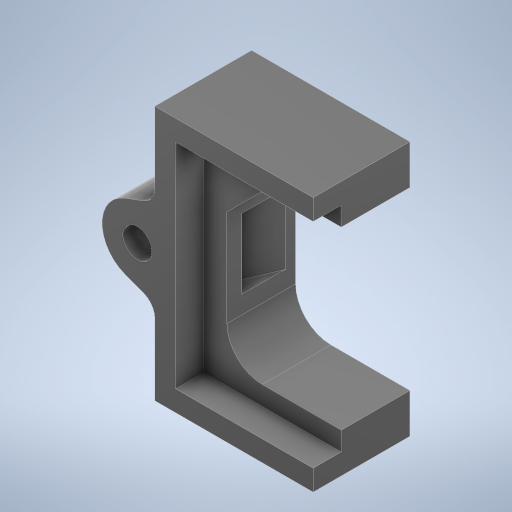
# Autodesk Inventor part: power_signal_socket_fixed2
Saved by Autodesk Inventor 2023 (Build 270158000, 158)
## iProperties
Created: 2023-09-07
Part Number: power_signal_socket_fixed2
Material: Acetal Resin, Black
Document SubType Name: Modeling
Designer: 310611102
Density: 1.425 g/cm^3
Appearance: Smooth - Black
Mass: 4.24079 g
Surface Area: 21.4214 cm^2
Volume: 2.97599 cm^3
Author: 310611102
Autodesk Inventor part; units mm, degrees
ref_plane "YZ Plane" through (0, 0, 0) normal (1, 0, 0) x (0, 1, 0)
ref_plane "XZ Plane" through (0, 0, 0) normal (0, 1, 0) x (-1, 0, 0)
ref_plane "XY Plane" through (0, 0, 0) normal (0, 0, 1) x (1, 0, 0)
sketch "Sketch2" plane through (0, 0, 0) normal (0, 0, 1) x (1, 0, 0)
  line L0 (-18, 14.5) -> (18, 14.5)
  line L1 (18, 14.5) -> (18, -14.5)
  line L2 (18, -14.5) -> (-18, -14.5)
  line L3 (-18, -14.5) -> (-18, 14.5)
  line L4 (-18, 14.5) -> (18, -14.5) construction
  line L5 (18, 14.5) -> (-18, -14.5) construction
  point P0 (0, 0)
  dimension "d0" = 29
  dimension "d1" = 36
  constraints: 12 end point, 2 midpoint, 2 parallel, 1 horizontal, 1 perpendicular
  measures "d0" distance of L0.end L1.end
  measures "d1" distance of L0.start L0.end
extrude "Extrusion1" add sketch "Sketch2" along normal blind 11
sketch "Sketch3" plane through (0, 0, 11) normal (0, 0, 1) x (1, 0, 0)
  line L0 (-15.65, 12.15) -> (15.65, 12.15)
  line L1 (15.65, 12.15) -> (15.65, -12.15)
  line L2 (15.65, -12.15) -> (-15.65, -12.15)
  line L3 (-15.65, -12.15) -> (-15.65, 12.15)
  line L4 (-15.65, 12.15) -> (15.65, -12.15) construction
  line L5 (15.65, 12.15) -> (-15.65, -12.15) construction
  point P0 (0, 0)
  dimension "d4" = 31.3
  dimension "d5" = 24.3
  constraints: 12 end point, 2 midpoint, 2 parallel, 1 horizontal, 1 perpendicular
  measures "d4" distance of L0.start L0.end
  measures "d5" distance of L0.end L1.end
extrude "Extrusion2" cut sketch "Sketch3" against normal blind 3.2
sketch "Sketch4" plane through (0, 0, 7.8) normal (0, 0, 1) x (1, 0, 0)
  line L0 (-8, 10) -> (8, 10)
  line L1 (13, 5) -> (13, -6)
  line L2 (9, -10) -> (-9, -10)
  line L3 (-13, -6) -> (-13, 5)
  line L4 (-13, 10) -> (13, -10) construction
  line L5 (13, 10) -> (-13, -10) construction
  line L6 (-13, 5) -> (-8, 10)
  line L7 (8, 10) -> (13, 5)
  arc A0 (-13, -6) -> (-9, -10) centre (-9, -6) ccw
  arc A1 (9, -10) -> (13, -6) centre (9, -6) ccw
  point P0 (0, 0)
  point P1 (-13, -4)
  point P2 (13, -4)
  dimension "d8" = 26
  dimension "d9" = 20
  dimension "d10" = 5
  dimension "d11" = 5
  dimension "d12" = 5
  dimension "d13" = 5
  dimension "d14" = 4
  constraints: 16 end point, 10 point on line, 4 point on circle, 4 tangent, 2 centre point, 2 midpoint, 2 parallel, 1 equal radius, 1 horizontal, 1 perpendicular
  measures "d8" distance of L4.start L5.start
  measures "d9" distance of L5.start L4.end
  measures "d10" distance of L3.end L4.start
  measures "d11" distance of L0.start L4.start
  measures "d12" distance of L0.end L5.start
  measures "d13" distance of L1.start L5.start
  measures "d14" radius of A0
extrude "Extrusion3" cut sketch "Sketch4" against normal through all
sketch "Sketch6" plane through (0, 0, 0) normal (0, 1, 0) x (-1, 0, 0)
  line L0 (13, 7.8) -> (13, 0) projected
  line L1 (13, 6.1) -> (15.1, 6.1)
  line L2 (15.1, 6.1) -> (13, 1.1)
  line L3 (13, 1.1) -> (13, 6.1)
  line L4 (15.65, 7.8) -> (-15.65, 7.8) projected
  line L5 (0, 0) -> (0, 10.1915) construction
  line L6 (-13, 7.8) -> (-13, 0)
  line L7 (-13, 6.1) -> (-15.1, 6.1)
  line L8 (-15.1, 6.1) -> (-13, 1.1)
  line L9 (-13, 1.1) -> (-13, 6.1)
  line L10 (-15.65, 7.8) -> (15.65, 7.8)
  dimension "d23" = 2.1
  dimension "d24" = 5
  dimension "d25" = 1.7
  constraints: 18 end point, 7 symmetric about line, 2 point on line, 1 horizontal, 1 perpendicular, 1 vertical
  measures "d23" distance of L1.start L1.end
  measures "d24" distance of L2.end L1.start
  measures "d25" distance between parallel lines of L4 L1
extrude "Extrusion5" cut sketch "Sketch6" along normal mid plane 8
sketch "Sketch7" plane through (0, 0, 11) normal (0, 0, 1) x (1, 0, 0)
  arc A0 (21.3831, -3.7533) -> (21.3831, 3.7533) centre (20, 0) ccw
  line L0 (21.3831, 3.7533) -> (18, 5)
  line L1 (18, 5) -> (18, -5)
  line L2 (13, 5) -> (13, -6) projected
  line L3 (18, -5) -> (21.3831, -3.7533)
  line L4 (0, 20.7674) -> (0, -20.7674) construction
  arc A1 (-21.3831, 3.7533) -> (-21.3831, -3.7533) centre (-20, 0) ccw
  line L5 (-21.3831, 3.7533) -> (-18, 5)
  line L6 (-18, 5) -> (-18, -5)
  line L7 (-18, -5) -> (-21.3831, -3.7533)
  line L8 (18, -14.5) -> (18, 14.5) construction
  circle A2 centre (20, 0) radius 1.65
  circle A3 centre (-20, 0) radius 1.65
  line L9 (0, 0) -> (1.9739, 0) construction
  dimension "d28" = 3.3
  dimension "d29" = 4
  dimension "d30" = 40
  dimension "d31" = 10
  constraints: 16 end point, 6 symmetric about line, 4 centre point, 4 point on circle, 2 coincident, 2 tangent, 1 horizontal, 1 horizontal alignment, 1 midpoint, 1 parallel, 1 point on line, 1 vertical, 3 other
  measures "d28" diameter of A2
  measures "d29" radius of A0
  measures "d30" distance of A1.centre A0.centre
  measures "d31" distance of L0.end L1.end
extrude "Extrusion6" add sketch "Sketch7" against normal up to surface (11 mm away)
fillet "Fillet1" radius 2 4 edges at (18, -5, 5.5) (18, 5, 5.5) (-18, 5, 5.5) (-18, -5, 5.5)
sketch "Sketch8" plane through (0, 0, 0) normal (1, 0, 0) x (0, 1, 0)
  line L0 (45.1511, -28.2394) -> (-45.1511, -28.2394)
  line L1 (-45.1511, -28.2394) -> (-45.1511, 28.2394)
  line L2 (-45.1511, 28.2394) -> (45.1511, 28.2394)
  line L3 (45.1511, 28.2394) -> (45.1511, -28.2394)
  line L4 (45.1511, -28.2394) -> (-45.1511, 28.2394) construction
  line L5 (-45.1511, -28.2394) -> (45.1511, 28.2394) construction
  point P0 (0, 0)
  constraints: 12 end point, 2 midpoint, 2 parallel, 1 horizontal, 1 perpendicular
extrude "Extrusion7" cut sketch "Sketch8" along normal through all
equation "\"d11\" = d10"
equation "\"d12\" = d10"
equation "\"d13\" = d12"
body "Solid1"
